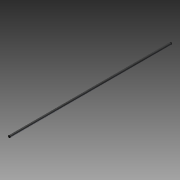
# Autodesk Inventor part: 2489 TR_1
Saved by Autodesk Inventor 2015 (Build 190159000, 159)
## iProperties
Company: Showman Fabricators
Created: 2016-05-10
Part Number: 2489 TR_1
Material: STEEL
Document SubType Name: Modeling
Designer: Josh
Density: 7.84905 g/cm^3
Sheet Metal Rule: Default
Appearance: STEEL MILL FINISH
Description: 3/8"-16 THREADED ROD, GRADE 5 OR BETTER
CNC: False
Author: Josh
Autodesk Inventor part; units mm, degrees
ref_plane "YZ Plane" through (0, 0, 0) normal (1, 0, 0) x (0, 1, 0)
ref_plane "XZ Plane" through (0, 0, 0) normal (0, 1, 0) x (-1, 0, 0)
ref_plane "XY Plane" through (0, 0, 0) normal (0, 0, 1) x (1, 0, 0)
sketch "CORNER RELIEF 3-8 BIT" plane through (0, 0, 0) normal (0, 0, 1) x (1, 0, 0)
  circle A0 centre (0, 0) radius 5.08
  point P0 (-5.08, 0)
  point P1 (0, 5.08)
  point P2 (5.08, 0)
  point P3 (0, -5.08)
  dimension "d6" = 45
  dimension "d0" = 10.16
  measures "d0" diameter of A0
sketch "Sketch2" plane through (0, 0, 0) normal (0, 0, 1) x (1, 0, 0)
  circle A0 centre (0, 0) radius 4.7625
  dimension "d1" = 9.525
  constraints: 1 centre point, 1 coincident
  measures "d1" diameter of A0
extrude "Extrusion1" add sketch "Sketch2" along normal mid plane 749.3
chamfer "Chamfer1" distance 0.7937 angle 45 2 edges at (-4.7625, 0, 374.65) (-4.7625, 0, -374.65)
thread "Thread1" size "3/8-16 UNC" class "2A" standard "ANSI Unified Screw Threads" full length
equation "\"PLY_1_2_THICK\" = 11.90752"
equation "\"PLY_3_4_THICK\" = 18.25752"
equation "\"WIG_WD_1_4_THICK\" = 4.7625"
equation "\"WIG_WD_3_8_THICK\" = 7.9375"
equation "\"MDF_1_2_THICK\" = 12"
equation "\"MDF_3_4_THICK\" = 18"
equation "\"BendRadius\" = Thickness"
equation "\"BendReliefWidth\" = Thickness"
equation "\"BendReliefDepth\" = 0.5 * Thickness"
equation "\"CornerReliefSize\" = 4 * Thickness"
equation "\"MinimumRemnant\" = 2 * Thickness"
equation "\"TransitionRadius\" = BendRadius"
equation "\"JacobiRadiusSize\" = BendRadius"
equation "\"GapSize\" = Thickness"
equation "\"Thickness\" = 3.048"
body "Solid1"
